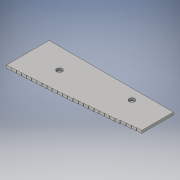
# Autodesk Inventor part: harry_potter_base
Saved by Autodesk Inventor 2016 (Build 200138000, 138)
## iProperties
Created: 2015-05-04
Part Number: harry_potter_base
Material: Generic
Document SubType Name: Modeling
Designer: Trevor
Density: 1 g/cm^3
Appearance: Default
Author: Trevor
Autodesk Inventor part; units mm, degrees
ref_plane "YZ Plane" through (0, 0, 0) normal (1, 0, 0) x (0, 1, 0)
ref_plane "XZ Plane" through (0, 0, 0) normal (0, 1, 0) x (-1, 0, 0)
ref_plane "XY Plane" through (0, 0, 0) normal (0, 0, 1) x (1, 0, 0)
sketch "Sketch1" plane through (0, 0, 0) normal (0, 1, 0) x (-1, 0, 0)
  line L0 (2.9308, 19.4492) -> (0, 19.4492)
  line L1 (0, 19.4492) -> (0, 0)
  line L2 (0, 0) -> (76.2, 0)
  line L3 (2.9308, 19.4492) -> (2.9308, 19.7994)
  line L4 (2.9308, 19.7994) -> (5.8615, 19.7994)
  line L5 (5.8615, 19.7994) -> (5.8615, 20.1396)
  line L6 (5.8615, 20.1396) -> (8.7923, 20.1396)
  line L7 (8.7923, 20.1396) -> (8.7923, 20.4702)
  line L8 (8.7923, 20.4702) -> (11.7231, 20.4702)
  line L9 (11.7231, 20.4702) -> (11.7231, 21.1032)
  line L10 (11.7231, 21.1032) -> (14.6538, 21.1032)
  line L11 (14.6538, 21.1032) -> (14.6538, 21.4063)
  line L12 (14.6538, 21.4063) -> (17.5846, 21.4063)
  line L13 (17.5846, 21.4063) -> (17.5846, 21.7008)
  line L14 (17.5846, 21.7008) -> (20.5154, 21.7008)
  line L15 (20.5154, 21.7008) -> (20.5154, 21.9869)
  line L16 (20.5154, 21.9869) -> (23.4462, 21.9869)
  line L17 (23.4462, 21.9869) -> (23.4462, 22.2648)
  line L18 (23.4462, 22.2648) -> (26.3769, 22.2648)
  line L19 (26.3769, 22.2648) -> (26.3769, 22.5348)
  line L20 (26.3769, 22.5348) -> (29.3077, 22.5348)
  line L21 (29.3077, 22.5348) -> (29.3077, 22.7972)
  line L22 (29.3077, 22.7972) -> (32.2385, 22.7972)
  line L23 (32.2385, 22.7972) -> (32.2385, 23.052)
  line L24 (32.2385, 23.052) -> (35.1692, 23.052)
  line L25 (35.1692, 23.052) -> (35.1692, 23.2997)
  line L26 (35.1692, 23.2997) -> (38.1, 23.2997)
  line L27 (38.1, 23.2997) -> (38.1, 23.7739)
  line L28 (38.1, 23.7739) -> (41.0308, 23.7739)
  line L29 (41.0308, 23.7739) -> (41.0308, 24.001)
  line L30 (41.0308, 24.001) -> (43.9615, 24.001)
  line L31 (43.9615, 24.001) -> (43.9615, 24.2216)
  line L32 (43.9615, 24.2216) -> (46.8923, 24.2216)
  line L33 (46.8923, 24.2216) -> (46.8923, 24.4359)
  line L34 (46.8923, 24.4359) -> (49.8231, 24.4359)
  line L35 (49.8231, 24.4359) -> (49.8231, 24.6441)
  line L36 (49.8231, 24.6441) -> (52.7538, 24.6441)
  line L37 (52.7538, 24.6441) -> (52.7538, 24.8464)
  line L38 (52.7538, 24.8464) -> (55.6846, 24.8464)
  line L39 (55.6846, 24.8464) -> (55.6846, 25.043)
  line L40 (55.6846, 25.043) -> (58.6154, 25.043)
  line L41 (58.6154, 25.043) -> (58.6154, 25.2339)
  line L42 (58.6154, 25.2339) -> (61.5462, 25.2339)
  line L43 (61.5462, 25.2339) -> (61.5462, 25.4194)
  line L44 (61.5462, 25.4194) -> (64.4769, 25.4194)
  line L45 (64.4769, 25.4194) -> (64.4769, 25.5996)
  line L46 (64.4769, 25.5996) -> (67.4077, 25.5996)
  line L47 (67.4077, 25.5996) -> (67.4077, 25.7747)
  line L48 (67.4077, 25.7747) -> (70.3385, 25.7747)
  line L49 (70.3385, 25.7747) -> (70.3385, 25.9448)
  line L50 (70.3385, 25.9448) -> (73.2692, 25.9448)
  line L51 (73.2692, 25.9448) -> (73.2692, 26.1101)
  line L52 (73.2692, 26.1101) -> (76.2, 26.1101)
  line L53 (76.2, 0) -> (76.2, 26.1101)
  circle A0 centre (19.05, 6.35) radius 1.7
  circle A1 centre (57.15, 12.7) radius 1.7
  constraints: 108 end point, 27 perpendicular, 26 parallel, 2 centre point, 1 equal radius
extrude "Extrusion1" add sketch "Sketch1" along normal blind 1.5875
body "Solid1"
